Autodesk Fusion 360 part; units mm, degrees
(part 4 of 5)
  spline S20 degree 5 poles (-21.545, 23.3234) (-21.543, 23.3196) (-21.5389, 23.3119) (-21.5325, 23.3007) (-21.5232, 23.286) (-21.5109, 23.2681) (-21.4979, 23.2506) (-21.4846, 23.2333) (-21.4711, 23.2161) (-21.4574, 23.199) (-21.4435, 23.182) (-21.4295, 23.165) (-21.4152, 23.1482) (-21.4006, 23.1316) (-21.3858, 23.1152) (-21.3706, 23.0989) (-21.3553, 23.0828) (-21.3397, 23.0668) (-21.324, 23.0509) (-21.3081, 23.0351) (-21.292, 23.0195) (-21.2758, 23.0039) (-21.2594, 22.9884) (-21.2428, 22.9731) (-21.2261, 22.9579) (-21.2092, 22.9427) (-21.1921, 22.9277) (-21.1748, 22.9128) (-21.1574, 22.8981) (-21.1399, 22.8834) (-21.1222, 22.8688) (-21.1044, 22.8543) (-21.0864, 22.8399) (-21.0683, 22.8256) (-21.05, 22.8114) (-21.0316, 22.7974) (-21.0131, 22.7834) (-20.9944, 22.7695) (-20.9756, 22.7557) (-20.9567, 22.742) (-20.9377, 22.7285) (-20.9185, 22.715) (-20.8992, 22.7016) (-20.8798, 22.6883) (-20.8602, 22.6751) (-20.8406, 22.662) (-20.8208, 22.649) (-20.8009, 22.6361) (-20.7808, 22.6233) (-20.7607, 22.6106) (-20.7405, 22.598) (-20.7201, 22.5854) (-20.6996, 22.573) (-20.679, 22.5607) (-20.6583, 22.5484) (-20.6375, 22.5363) (-20.6166, 22.5243) (-20.5956, 22.5123) (-20.5744, 22.5004) (-20.5532, 22.4887) (-20.5319, 22.477) (-20.5104, 22.4654) (-20.4889, 22.454) (-20.4672, 22.4426) (-20.4455, 22.4313) (-20.4237, 22.4201) (-20.4017, 22.409) (-20.3797, 22.398) (-20.3575, 22.3871) (-20.3353, 22.3763) (-20.313, 22.3655) (-20.295, 22.357) (-20.2815, 22.3507) (-20.2725, 22.3465) (-20.268, 22.3444) knots 0 0 0 0 0 0 0.01428571 0.02857143 0.04285714 0.05714286 0.07142857 0.08571429 0.1 0.11428571 0.12857143 0.14285714 0.15714286 0.17142857 0.18571429 0.2 0.21428571 0.22857143 0.24285714 0.25714286 0.27142857 0.28571429 0.3 0.31428571 0.32857143 0.34285714 0.35714286 0.37142857 0.38571429 0.4 0.41428571 0.42857143 0.44285714 0.45714286 0.47142857 0.48571429 0.5 0.51428571 0.52857143 0.54285714 0.55714286 0.57142857 0.58571429 0.6 0.61428571 0.62857143 0.64285714 0.65714286 0.67142857 0.68571429 0.7 0.71428571 0.72857143 0.74285714 0.75714286 0.77142857 0.78571429 0.8 0.81428571 0.82857143 0.84285714 0.85714286 0.87142857 0.88571429 0.9 0.91428571 0.92857143 0.94285714 0.95714286 0.97142857 0.98571429 1 1 1 1 1 1
  line L23 (-21.545, 23.3234) -> (-21.677, 23.5776)
  arc A42 (-21.677, 23.5776) -> (-22.3193, 23.806) centre (-22.1207, 23.3471) ccw
  arc A43 (-22.5157, 23.7247) -> (-22.3193, 23.806) centre (-25, 30) ccw
  arc A44 (-22.5157, 23.7247) -> (-22.8084, 23.1089) centre (-22.3317, 23.2598) ccw
  line L24 (-22.8084, 23.1089) -> (-22.722, 22.8359)
  spline S21 degree 5 poles (-22.722, 22.8359) (-22.7207, 22.8318) (-22.7182, 22.8235) (-22.7148, 22.8109) (-22.7109, 22.794) (-22.707, 22.7727) (-22.7038, 22.7511) (-22.701, 22.7295) (-22.6984, 22.7077) (-22.696, 22.6859) (-22.6937, 22.6641) (-22.6917, 22.6422) (-22.6899, 22.6202) (-22.6885, 22.5982) (-22.6874, 22.5761) (-22.6866, 22.5539) (-22.686, 22.5316) (-22.6857, 22.5093) (-22.6856, 22.4869) (-22.6857, 22.4645) (-22.6859, 22.4421) (-22.6864, 22.4196) (-22.6871, 22.3971) (-22.6879, 22.3745) (-22.689, 22.3519) (-22.6903, 22.3292) (-22.6918, 22.3065) (-22.6934, 22.2838) (-22.6953, 22.2611) (-22.6973, 22.2383) (-22.6995, 22.2154) (-22.7018, 22.1926) (-22.7044, 22.1697) (-22.7071, 22.1468) (-22.71, 22.1239) (-22.713, 22.1009) (-22.7162, 22.0779) (-22.7196, 22.0549) (-22.7232, 22.0319) (-22.7269, 22.0088) (-22.7307, 21.9858) (-22.7348, 21.9627) (-22.7389, 21.9395) (-22.7433, 21.9164) (-22.7478, 21.8933) (-22.7524, 21.8701) (-22.7572, 21.8469) (-22.7622, 21.8237) (-22.7673, 21.8005) (-22.7725, 21.7773) (-22.7779, 21.754) (-22.7835, 21.7308) (-22.7892, 21.7075) (-22.795, 21.6842) (-22.801, 21.6609) (-22.8071, 21.6376) (-22.8134, 21.6143) (-22.8198, 21.591) (-22.8264, 21.5677) (-22.833, 21.5443) (-22.8399, 21.521) (-22.8469, 21.4977) (-22.854, 21.4743) (-22.8612, 21.451) (-22.8686, 21.4276) (-22.8762, 21.4042) (-22.8838, 21.3809) (-22.8916, 21.3575) (-22.8996, 21.3341) (-22.9076, 21.3108) (-22.9158, 21.2874) (-22.9225, 21.2687) (-22.9276, 21.2547) (-22.931, 21.2453) (-22.9327, 21.2406) knots 0 0 0 0 0 0 0.01428571 0.02857143 0.04285714 0.05714286 0.07142857 0.08571429 0.1 0.11428571 0.12857143 0.14285714 0.15714286 0.17142857 0.18571429 0.2 0.21428571 0.22857143 0.24285714 0.25714286 0.27142857 0.28571429 0.3 0.31428571 0.32857143 0.34285714 0.35714286 0.37142857 0.38571429 0.4 0.41428571 0.42857143 0.44285714 0.45714286 0.47142857 0.48571429 0.5 0.51428571 0.52857143 0.54285714 0.55714286 0.57142857 0.58571429 0.6 0.61428571 0.62857143 0.64285714 0.65714286 0.67142857 0.68571429 0.7 0.71428571 0.72857143 0.74285714 0.75714286 0.77142857 0.78571429 0.8 0.81428571 0.82857143 0.84285714 0.85714286 0.87142857 0.88571429 0.9 0.91428571 0.92857143 0.94285714 0.95714286 0.97142857 0.98571429 1 1 1 1 1 1
  arc A45 (-23.5579, 21.1163) -> (-22.9327, 21.2406) centre (-25, 30) ccw
  spline S22 degree 5 poles (-24.363, 22.5095) (-24.3627, 22.5052) (-24.3618, 22.4965) (-24.3601, 22.4837) (-24.3572, 22.4666) (-24.3527, 22.4453) (-24.3474, 22.4242) (-24.3417, 22.4031) (-24.3358, 22.382) (-24.3297, 22.361) (-24.3234, 22.3399) (-24.3169, 22.3189) (-24.3101, 22.298) (-24.303, 22.277) (-24.2956, 22.2562) (-24.2878, 22.2354) (-24.2798, 22.2146) (-24.2715, 22.1939) (-24.2631, 22.1731) (-24.2544, 22.1525) (-24.2456, 22.1318) (-24.2366, 22.1112) (-24.2274, 22.0907) (-24.2179, 22.0702) (-24.2083, 22.0497) (-24.1984, 22.0293) (-24.1884, 22.0089) (-24.1781, 21.9885) (-24.1677, 21.9682) (-24.1571, 21.9479) (-24.1464, 21.9276) (-24.1355, 21.9074) (-24.1244, 21.8873) (-24.1131, 21.8671) (-24.1016, 21.8471) (-24.09, 21.827) (-24.0783, 21.807) (-24.0663, 21.787) (-24.0542, 21.7671) (-24.042, 21.7472) (-24.0296, 21.7274) (-24.017, 21.7076) (-24.0043, 21.6878) (-23.9915, 21.6681) (-23.9785, 21.6485) (-23.9653, 21.6288) (-23.952, 21.6092) (-23.9385, 21.5897) (-23.925, 21.5702) (-23.9112, 21.5508) (-23.8973, 21.5313) (-23.8833, 21.512) (-23.8691, 21.4927) (-23.8548, 21.4734) (-23.8404, 21.4542) (-23.8258, 21.435) (-23.8111, 21.4159) (-23.7963, 21.3968) (-23.7813, 21.3777) (-23.7662, 21.3587) (-23.7509, 21.3398) (-23.7355, 21.3209) (-23.72, 21.302) (-23.7044, 21.2832) (-23.6886, 21.2645) (-23.6727, 21.2458) (-23.6567, 21.2271) (-23.6405, 21.2085) (-23.6243, 21.19) (-23.6079, 21.1715) (-23.5913, 21.153) (-23.578, 21.1383) (-23.568, 21.1273) (-23.5613, 21.12) (-23.5579, 21.1163) knots 0 0 0 0 0 0 0.01428571 0.02857143 0.04285714 0.05714286 0.07142857 0.08571429 0.1 0.11428571 0.12857143 0.14285714 0.15714286 0.17142857 0.18571429 0.2 0.21428571 0.22857143 0.24285714 0.25714286 0.27142857 0.28571429 0.3 0.31428571 0.32857143 0.34285714 0.35714286 0.37142857 0.38571429 0.4 0.41428571 0.42857143 0.44285714 0.45714286 0.47142857 0.48571429 0.5 0.51428571 0.52857143 0.54285714 0.55714286 0.57142857 0.58571429 0.6 0.61428571 0.62857143 0.64285714 0.65714286 0.67142857 0.68571429 0.7 0.71428571 0.72857143 0.74285714 0.75714286 0.77142857 0.78571429 0.8 0.81428571 0.82857143 0.84285714 0.85714286 0.87142857 0.88571429 0.9 0.91428571 0.92857143 0.94285714 0.95714286 0.97142857 0.98571429 1 1 1 1 1 1
  line L25 (-24.363, 22.5095) -> (-24.3877, 22.7948)
  arc A46 (-24.3877, 22.7948) -> (-24.8937, 23.2516) centre (-24.8858, 22.7517) ccw
  arc A47 (-25.1063, 23.2516) -> (-24.8937, 23.2516) centre (-25, 30) ccw
  arc A48 (-25.1063, 23.2516) -> (-25.6123, 22.7948) centre (-25.1142, 22.7517) ccw
  line L26 (-25.6123, 22.7948) -> (-25.637, 22.5095)
  spline S23 degree 5 poles (-25.637, 22.5095) (-25.6373, 22.5052) (-25.6382, 22.4965) (-25.6399, 22.4837) (-25.6428, 22.4666) (-25.6473, 22.4453) (-25.6526, 22.4242) (-25.6583, 22.4031) (-25.6642, 22.382) (-25.6703, 22.361) (-25.6766, 22.3399) (-25.6831, 22.3189) (-25.6899, 22.298) (-25.697, 22.277) (-25.7044, 22.2562) (-25.7122, 22.2354) (-25.7202, 22.2146) (-25.7285, 22.1939) (-25.7369, 22.1731) (-25.7456, 22.1525) (-25.7544, 22.1318) (-25.7634, 22.1112) (-25.7726, 22.0907) (-25.7821, 22.0702) (-25.7917, 22.0497) (-25.8016, 22.0293) (-25.8116, 22.0089) (-25.8219, 21.9885) (-25.8323, 21.9682) (-25.8429, 21.9479) (-25.8536, 21.9276) (-25.8645, 21.9074) (-25.8756, 21.8873) (-25.8869, 21.8671) (-25.8984, 21.8471) (-25.91, 21.827) (-25.9217, 21.807) (-25.9337, 21.787) (-25.9458, 21.7671) (-25.958, 21.7472) (-25.9704, 21.7274) (-25.983, 21.7076) (-25.9957, 21.6878) (-26.0085, 21.6681) (-26.0215, 21.6485) (-26.0347, 21.6288) (-26.048, 21.6092) (-26.0615, 21.5897) (-26.075, 21.5702) (-26.0888, 21.5508) (-26.1027, 21.5313) (-26.1167, 21.512) (-26.1309, 21.4927) (-26.1452, 21.4734) (-26.1596, 21.4542) (-26.1742, 21.435) (-26.1889, 21.4159) (-26.2037, 21.3968) (-26.2187, 21.3777) (-26.2338, 21.3587) (-26.2491, 21.3398) (-26.2645, 21.3209) (-26.28, 21.302) (-26.2956, 21.2832) (-26.3114, 21.2645) (-26.3273, 21.2458) (-26.3433, 21.2271) (-26.3595, 21.2085) (-26.3757, 21.19) (-26.3921, 21.1715) (-26.4087, 21.153) (-26.422, 21.1383) (-26.432, 21.1273) (-26.4387, 21.12) (-26.4421, 21.1163) knots 0 0 0 0 0 0 0.01428571 0.02857143 0.04285714 0.05714286 0.07142857 0.08571429 0.1 0.11428571 0.12857143 0.14285714 0.15714286 0.17142857 0.18571429 0.2 0.21428571 0.22857143 0.24285714 0.25714286 0.27142857 0.28571429 0.3 0.31428571 0.32857143 0.34285714 0.35714286 0.37142857 0.38571429 0.4 0.41428571 0.42857143 0.44285714 0.45714286 0.47142857 0.48571429 0.5 0.51428571 0.52857143 0.54285714 0.55714286 0.57142857 0.58571429 0.6 0.61428571 0.62857143 0.64285714 0.65714286 0.67142857 0.68571429 0.7 0.71428571 0.72857143 0.74285714 0.75714286 0.77142857 0.78571429 0.8 0.81428571 0.82857143 0.84285714 0.85714286 0.87142857 0.88571429 0.9 0.91428571 0.92857143 0.94285714 0.95714286 0.97142857 0.98571429 1 1 1 1 1 1
  arc A49 (-27.0673, 21.2406) -> (-26.4421, 21.1163) centre (-25, 30) ccw
  spline S24 degree 5 poles (-27.278, 22.8359) (-27.2793, 22.8318) (-27.2818, 22.8235) (-27.2852, 22.8109) (-27.2891, 22.794) (-27.293, 22.7727) (-27.2962, 22.7511) (-27.299, 22.7295) (-27.3016, 22.7077) (-27.304, 22.6859) (-27.3063, 22.6641) (-27.3083, 22.6422) (-27.3101, 22.6202) (-27.3115, 22.5982) (-27.3126, 22.5761) (-27.3134, 22.5539) (-27.314, 22.5316) (-27.3143, 22.5093) (-27.3144, 22.4869) (-27.3143, 22.4645) (-27.3141, 22.4421) (-27.3136, 22.4196) (-27.3129, 22.3971) (-27.3121, 22.3745) (-27.311, 22.3519) (-27.3097, 22.3292) (-27.3082, 22.3065) (-27.3066, 22.2838) (-27.3047, 22.2611) (-27.3027, 22.2383) (-27.3005, 22.2154) (-27.2982, 22.1926) (-27.2956, 22.1697) (-27.2929, 22.1468) (-27.29, 22.1239) (-27.287, 22.1009) (-27.2838, 22.0779) (-27.2804, 22.0549) (-27.2768, 22.0319) (-27.2731, 22.0088) (-27.2693, 21.9858) (-27.2652, 21.9627) (-27.2611, 21.9395) (-27.2567, 21.9164) (-27.2522, 21.8933) (-27.2476, 21.8701) (-27.2428, 21.8469) (-27.2378, 21.8237) (-27.2327, 21.8005) (-27.2275, 21.7773) (-27.2221, 21.754) (-27.2165, 21.7308) (-27.2108, 21.7075) (-27.205, 21.6842) (-27.199, 21.6609) (-27.1929, 21.6376) (-27.1866, 21.6143) (-27.1802, 21.591) (-27.1736, 21.5677) (-27.167, 21.5443) (-27.1601, 21.521) (-27.1531, 21.4977) (-27.146, 21.4743) (-27.1388, 21.451) (-27.1314, 21.4276) (-27.1238, 21.4042) (-27.1162, 21.3809) (-27.1084, 21.3575) (-27.1004, 21.3341) (-27.0924, 21.3108) (-27.0842, 21.2874) (-27.0775, 21.2687) (-27.0724, 21.2547) (-27.069, 21.2453) (-27.0673, 21.2406) knots 0 0 0 0 0 0 0.01428571 0.02857143 0.04285714 0.05714286 0.07142857 0.08571429 0.1 0.11428571 0.12857143 0.14285714 0.15714286 0.17142857 0.18571429 0.2 0.21428571 0.22857143 0.24285714 0.25714286 0.27142857 0.28571429 0.3 0.31428571 0.32857143 0.34285714 0.35714286 0.37142857 0.38571429 0.4 0.41428571 0.42857143 0.44285714 0.45714286 0.47142857 0.48571429 0.5 0.51428571 0.52857143 0.54285714 0.55714286 0.57142857 0.58571429 0.6 0.61428571 0.62857143 0.64285714 0.65714286 0.67142857 0.68571429 0.7 0.71428571 0.72857143 0.74285714 0.75714286 0.77142857 0.78571429 0.8 0.81428571 0.82857143 0.84285714 0.85714286 0.87142857 0.88571429 0.9 0.91428571 0.92857143 0.94285714 0.95714286 0.97142857 0.98571429 1 1 1 1 1 1
  line L27 (-27.278, 22.8359) -> (-27.1916, 23.1089)
  arc A50 (-27.1916, 23.1089) -> (-27.4843, 23.7247) centre (-27.6683, 23.2598) ccw
  arc A51 (-27.6807, 23.806) -> (-27.4843, 23.7247) centre (-25, 30) ccw
  arc A52 (-27.6807, 23.806) -> (-28.323, 23.5776) centre (-27.8793, 23.3471) ccw
  line L28 (-28.323, 23.5776) -> (-28.455, 23.3234)
  spline S25 degree 5 poles (-28.455, 23.3234) (-28.457, 23.3196) (-28.4611, 23.3119) (-28.4675, 23.3007) (-28.4768, 23.286) (-28.4891, 23.2681) (-28.5021, 23.2506) (-28.5154, 23.2333) (-28.5289, 23.2161) (-28.5426, 23.199) (-28.5565, 23.182) (-28.5705, 23.165) (-28.5848, 23.1482) (-28.5994, 23.1316) (-28.6142, 23.1152) (-28.6294, 23.0989) (-28.6447, 23.0828) (-28.6603, 23.0668) (-28.676, 23.0509) (-28.6919, 23.0351) (-28.708, 23.0195) (-28.7242, 23.0039) (-28.7406, 22.9884) (-28.7572, 22.9731) (-28.7739, 22.9579) (-28.7908, 22.9427) (-28.8079, 22.9277) (-28.8252, 22.9128) (-28.8426, 22.8981) (-28.8601, 22.8834) (-28.8778, 22.8688) (-28.8956, 22.8543) (-28.9136, 22.8399) (-28.9317, 22.8256) (-28.95, 22.8114) (-28.9684, 22.7974) (-28.9869, 22.7834) (-29.0056, 22.7695) (-29.0244, 22.7557) (-29.0433, 22.742) (-29.0623, 22.7285) (-29.0815, 22.715) (-29.1008, 22.7016) (-29.1202, 22.6883) (-29.1398, 22.6751) (-29.1594, 22.662) (-29.1792, 22.649) (-29.1991, 22.6361) (-29.2192, 22.6233) (-29.2393, 22.6106) (-29.2595, 22.598) (-29.2799, 22.5854) (-29.3004, 22.573) (-29.321, 22.5607) (-29.3417, 22.5484) (-29.3625, 22.5363) (-29.3834, 22.5243) (-29.4044, 22.5123) (-29.4256, 22.5004) (-29.4468, 22.4887) (-29.4681, 22.477) (-29.4896, 22.4654) (-29.5111, 22.454) (-29.5328, 22.4426) (-29.5545, 22.4313) (-29.5763, 22.4201) (-29.5983, 22.409) (-29.6203, 22.398) (-29.6425, 22.3871) (-29.6647, 22.3763) (-29.687, 22.3655) (-29.705, 22.357) (-29.7185, 22.3507) (-29.7275, 22.3465) (-29.732, 22.3444) knots 0 0 0 0 0 0 0.01428571 0.02857143 0.04285714 0.05714286 0.07142857 0.08571429 0.1 0.11428571 0.12857143 0.14285714 0.15714286 0.17142857 0.18571429 0.2 0.21428571 0.22857143 0.24285714 0.25714286 0.27142857 0.28571429 0.3 0.31428571 0.32857143 0.34285714 0.35714286 0.37142857 0.38571429 0.4 0.41428571 0.42857143 0.44285714 0.45714286 0.47142857 0.48571429 0.5 0.51428571 0.52857143 0.54285714 0.55714286 0.57142857 0.58571429 0.6 0.61428571 0.62857143 0.64285714 0.65714286 0.67142857 0.68571429 0.7 0.71428571 0.72857143 0.74285714 0.75714286 0.77142857 0.78571429 0.8 0.81428571 0.82857143 0.84285714 0.85714286 0.87142857 0.88571429 0.9 0.91428571 0.92857143 0.94285714 0.95714286 0.97142857 0.98571429 1 1 1 1 1 1
  arc A53 (-30.262, 22.6985) -> (-29.732, 22.3444) centre (-25, 30) ccw
  spline S26 degree 5 poles (-29.8462, 24.253) (-29.849, 24.2497) (-29.8545, 24.243) (-29.8624, 24.2327) (-29.8724, 24.2186) (-29.8842, 24.2003) (-29.8954, 24.1816) (-29.9063, 24.1627) (-29.917, 24.1436) (-29.9276, 24.1244) (-29.938, 24.1051) (-29.9483, 24.0856) (-29.9583, 24.066) (-29.9681, 24.0462) (-29.9776, 24.0262) (-29.9868, 24.006) (-29.9959, 23.9856) (-30.0047, 23.9651) (-30.0133, 23.9445) (-30.0218, 23.9238) (-30.0302, 23.9029) (-30.0384, 23.882) (-30.0464, 23.8609) (-30.0542, 23.8397) (-30.0619, 23.8184) (-30.0694, 23.797) (-30.0767, 23.7755) (-30.0838, 23.7539) (-30.0909, 23.7321) (-30.0977, 23.7103) (-30.1044, 23.6884) (-30.111, 23.6664) (-30.1174, 23.6443) (-30.1237, 23.6221) (-30.1298, 23.5998) (-30.1357, 23.5774) (-30.1416, 23.5549) (-30.1472, 23.5324) (-30.1528, 23.5097) (-30.1582, 23.487) (-30.1634, 23.4642) (-30.1686, 23.4413) (-30.1735, 23.4184) (-30.1784, 23.3953) (-30.1831, 23.3722) (-30.1877, 23.349) (-30.1921, 23.3258) (-30.1964, 23.3025) (-30.2006, 23.2791) (-30.2046, 23.2556) (-30.2085, 23.2321) (-30.2123, 23.2084) (-30.216, 23.1848) (-30.2195, 23.161) (-30.2229, 23.1372) (-30.2261, 23.1134) (-30.2292, 23.0894) (-30.2322, 23.0654) (-30.2351, 23.0414) (-30.2378, 23.0172) (-30.2405, 22.9931) (-30.2429, 22.9688) (-30.2453, 22.9445) (-30.2475, 22.9202) (-30.2497, 22.8958) (-30.2516, 22.8713) (-30.2535, 22.8468) (-30.2552, 22.8222) (-30.2568, 22.7976) (-30.2583, 22.7729) (-30.2597, 22.7482) (-30.2607, 22.7283) (-30.2614, 22.7135) (-30.2618, 22.7035) (-30.262, 22.6985) knots 0 0 0 0 0 0 0.01428571 0.02857143 0.04285714 0.05714286 0.07142857 0.08571429 0.1 0.11428571 0.12857143 0.14285714 0.15714286 0.17142857 0.18571429 0.2 0.21428571 0.22857143 0.24285714 0.25714286 0.27142857 0.28571429 0.3 0.31428571 0.32857143 0.34285714 0.35714286 0.37142857 0.38571429 0.4 0.41428571 0.42857143 0.44285714 0.45714286 0.47142857 0.48571429 0.5 0.51428571 0.52857143 0.54285714 0.55714286 0.57142857 0.58571429 0.6 0.61428571 0.62857143 0.64285714 0.65714286 0.67142857 0.68571429 0.7 0.71428571 0.72857143 0.74285714 0.75714286 0.77142857 0.78571429 0.8 0.81428571 0.82857143 0.84285714 0.85714286 0.87142857 0.88571429 0.9 0.91428571 0.92857143 0.94285714 0.95714286 0.97142857 0.98571429 1 1 1 1 1 1
  line L29 (-29.8462, 24.253) -> (-29.6619, 24.4722)
  arc A54 (-29.6619, 24.4722) -> (-29.6967, 25.153) centre (-30.0446, 24.794) ccw
  arc A55 (-29.847, 25.3033) -> (-29.6967, 25.153) centre (-25, 30) ccw
  arc A56 (-29.847, 25.3033) -> (-30.5278, 25.3381) centre (-30.206, 24.9554) ccw
  line L30 (-30.5278, 25.3381) -> (-30.747, 25.1538)
  spline S27 degree 5 poles (-30.747, 25.1538) (-30.7503, 25.151) (-30.757, 25.1455) (-30.7673, 25.1376) (-30.7814, 25.1276) (-30.7997, 25.1158) (-30.8184, 25.1046) (-30.8373, 25.0937) (-30.8564, 25.083) (-30.8756, 25.0724) (-30.8949, 25.062) (-30.9144, 25.0517) (-30.934, 25.0417) (-30.9538, 25.0319) (-30.9738, 25.0224) (-30.994, 25.0132) (-31.0144, 25.0041) (-31.0349, 24.9953) (-31.0555, 24.9867) (-31.0762, 24.9782) (-31.0971, 24.9698) (-31.118, 24.9616) (-31.1391, 24.9536) (-31.1603, 24.9458) (-31.1816, 24.9381) (-31.203, 24.9306) (-31.2245, 24.9233) (-31.2461, 24.9162) (-31.2679, 24.9091) (-31.2897, 24.9023) (-31.3116, 24.8956) (-31.3336, 24.889) (-31.3557, 24.8826) (-31.3779, 24.8763) (-31.4002, 24.8702) (-31.4226, 24.8643) (-31.4451, 24.8584) (-31.4676, 24.8528) (-31.4903, 24.8472) (-31.513, 24.8418) (-31.5358, 24.8366) (-31.5587, 24.8314) (-31.5816, 24.8265) (-31.6047, 24.8216) (-31.6278, 24.8169) (-31.651, 24.8123) (-31.6742, 24.8079) (-31.6975, 24.8036) (-31.7209, 24.7994) (-31.7444, 24.7954) (-31.7679, 24.7915) (-31.7916, 24.7877) (-31.8152, 24.784) (-31.839, 24.7805) (-31.8628, 24.7771) (-31.8866, 24.7739) (-31.9106, 24.7708) (-31.9346, 24.7678) (-31.9586, 24.7649) (-31.9828, 24.7622) (-32.0069, 24.7595) (-32.0312, 24.7571) (-32.0555, 24.7547) (-32.0798, 24.7525) (-32.1042, 24.7503) (-32.1287, 24.7484) (-32.1532, 24.7465) (-32.1778, 24.7448) (-32.2024, 24.7432) (-32.2271, 24.7417) (-32.2518, 24.7403) (-32.2717, 24.7393) (-32.2865, 24.7386) (-32.2965, 24.7382) (-32.3015, 24.738) knots 0 0 0 0 0 0 0.01428571 0.02857143 0.04285714 0.05714286 0.07142857 0.08571429 0.1 0.11428571 0.12857143 0.14285714 0.15714286 0.17142857 0.18571429 0.2 0.21428571 0.22857143 0.24285714 0.25714286 0.27142857 0.28571429 0.3 0.31428571 0.32857143 0.34285714 0.35714286 0.37142857 0.38571429 0.4 0.41428571 0.42857143 0.44285714 0.45714286 0.47142857 0.48571429 0.5 0.51428571 0.52857143 0.54285714 0.55714286 0.57142857 0.58571429 0.6 0.61428571 0.62857143 0.64285714 0.65714286 0.67142857 0.68571429 0.7 0.71428571 0.72857143 0.74285714 0.75714286 0.77142857 0.78571429 0.8 0.81428571 0.82857143 0.84285714 0.85714286 0.87142857 0.88571429 0.9 0.91428571 0.92857143 0.94285714 0.95714286 0.97142857 0.98571429 1 1 1 1 1 1
  arc A57 (-32.6556, 25.268) -> (-32.3015, 24.738) centre (-25, 30) ccw
  spline S28 degree 5 poles (-31.6766, 26.545) (-31.6804, 26.543) (-31.6881, 26.5389) (-31.6993, 26.5325) (-31.714, 26.5232) (-31.7319, 26.5109) (-31.7494, 26.4979) (-31.7667, 26.4846) (-31.7839, 26.4711) (-31.801, 26.4574) (-31.818, 26.4435) (-31.835, 26.4295) (-31.8518, 26.4152) (-31.8684, 26.4006) (-31.8848, 26.3858) (-31.9011, 26.3706) (-31.9172, 26.3553) (-31.9332, 26.3397) (-31.9491, 26.324) (-31.9649, 26.3081) (-31.9805, 26.292) (-31.9961, 26.2758) (-32.0116, 26.2594) (-32.0269, 26.2428) (-32.0421, 26.2261) (-32.0573, 26.2092) (-32.0723, 26.1921) (-32.0872, 26.1748) (-32.1019, 26.1574) (-32.1166, 26.1399) (-32.1312, 26.1222) (-32.1457, 26.1044) (-32.1601, 26.0864) (-32.1744, 26.0683) (-32.1886, 26.05) (-32.2026, 26.0316) (-32.2166, 26.0131) (-32.2305, 25.9944) (-32.2443, 25.9756) (-32.258, 25.9567) (-32.2715, 25.9377) (-32.285, 25.9185) (-32.2984, 25.8992) (-32.3117, 25.8798) (-32.3249, 25.8602) (-32.338, 25.8406) (-32.351, 25.8208) (-32.3639, 25.8009) (-32.3767, 25.7808) (-32.3894, 25.7607) (-32.402, 25.7405) (-32.4146, 25.7201) (-32.427, 25.6996) (-32.4393, 25.679) (-32.4516, 25.6583) (-32.4637, 25.6375) (-32.4757, 25.6166) (-32.4877, 25.5956) (-32.4996, 25.5744) (-32.5113, 25.5532) (-32.523, 25.5319) (-32.5346, 25.5104) (-32.546, 25.4889) (-32.5574, 25.4672) (-32.5687, 25.4455) (-32.5799, 25.4237) (-32.591, 25.4017) (-32.602, 25.3797) (-32.6129, 25.3575) (-32.6237, 25.3353) (-32.6345, 25.313) (-32.643, 25.295) (-32.6493, 25.2815) (-32.6535, 25.2725) (-32.6556, 25.268) knots 0 0 0 0 0 0 0.01428571 0.02857143 0.04285714 0.05714286 0.07142857 0.08571429 0.1 0.11428571 0.12857143 0.14285714 0.15714286 0.17142857 0.18571429 0.2 0.21428571 0.22857143 0.24285714 0.25714286 0.27142857 0.28571429 0.3 0.31428571 0.32857143 0.34285714 0.35714286 0.37142857 0.38571429 0.4 0.41428571 0.42857143 0.44285714 0.45714286 0.47142857 0.48571429 0.5 0.51428571 0.52857143 0.54285714 0.55714286 0.57142857 0.58571429 0.6 0.61428571 0.62857143 0.64285714 0.65714286 0.67142857 0.68571429 0.7 0.71428571 0.72857143 0.74285714 0.75714286 0.77142857 0.78571429 0.8 0.81428571 0.82857143 0.84285714 0.85714286 0.87142857 0.88571429 0.9 0.91428571 0.92857143 0.94285714 0.95714286 0.97142857 0.98571429 1 1 1 1 1 1
  line L31 (-31.6766, 26.545) -> (-31.4224, 26.677)
  arc A58 (-31.4224, 26.677) -> (-31.194, 27.3193) centre (-31.6529, 27.1207) ccw
  arc A59 (-31.2753, 27.5157) -> (-31.194, 27.3193) centre (-25, 30) ccw
  arc A60 (-31.2753, 27.5157) -> (-31.8911, 27.8084) centre (-31.7402, 27.3317) ccw
  line L32 (-31.8911, 27.8084) -> (-32.1641, 27.722)
  spline S29 degree 5 poles (-32.1641, 27.722) (-32.1682, 27.7207) (-32.1765, 27.7182) (-32.1891, 27.7148) (-32.206, 27.7109) (-32.2273, 27.707) (-32.2489, 27.7038) (-32.2705, 27.701) (-32.2923, 27.6984) (-32.3141, 27.696) (-32.3359, 27.6937) (-32.3578, 27.6917) (-32.3798, 27.6899) (-32.4018, 27.6885) (-32.4239, 27.6874) (-32.4461, 27.6866) (-32.4684, 27.686) (-32.4907, 27.6857) (-32.5131, 27.6856) (-32.5355, 27.6857) (-32.5579, 27.6859) (-32.5804, 27.6864) (-32.6029, 27.6871) (-32.6255, 27.6879) (-32.6481, 27.689) (-32.6708, 27.6903) (-32.6935, 27.6918) (-32.7162, 27.6934) (-32.7389, 27.6953) (-32.7617, 27.6973) (-32.7846, 27.6995) (-32.8074, 27.7018) (-32.8303, 27.7044) (-32.8532, 27.7071) (-32.8761, 27.71) (-32.8991, 27.713) (-32.9221, 27.7162) (-32.9451, 27.7196) (-32.9681, 27.7232) (-32.9912, 27.7269) (-33.0142, 27.7307) (-33.0373, 27.7348) (-33.0605, 27.7389) (-33.0836, 27.7433) (-33.1067, 27.7478) (-33.1299, 27.7524) (-33.1531, 27.7572) (-33.1763, 27.7622) (-33.1995, 27.7673) (-33.2227, 27.7725) (-33.246, 27.7779) (-33.2692, 27.7835) (-33.2925, 27.7892) (-33.3158, 27.795) (-33.3391, 27.801) (-33.3624, 27.8071) (-33.3857, 27.8134) (-33.409, 27.8198) (-33.4323, 27.8264) (-33.4557, 27.833) (-33.479, 27.8399) (-33.5023, 27.8469) (-33.5257, 27.854) (-33.549, 27.8612) (-33.5724, 27.8686) (-33.5958, 27.8762) (-33.6191, 27.8838) (-33.6425, 27.8916) (-33.6659, 27.8996) (-33.6892, 27.9076) (-33.7126, 27.9158) (-33.7313, 27.9225) (-33.7453, 27.9276) (-33.7547, 27.931) (-33.7594, 27.9327) knots 0 0 0 0 0 0 0.01428571 0.02857143 0.04285714 0.05714286 0.07142857 0.08571429 0.1 0.11428571 0.12857143 0.14285714 0.15714286 0.17142857 0.18571429 0.2 0.21428571 0.22857143 0.24285714 0.25714286 0.27142857 0.28571429 0.3 0.31428571 0.32857143 0.34285714 0.35714286 0.37142857 0.38571429 0.4 0.41428571 0.42857143 0.44285714 0.45714286 0.47142857 0.48571429 0.5 0.51428571 0.52857143 0.54285714 0.55714286 0.57142857 0.58571429 0.6 0.61428571 0.62857143 0.64285714 0.65714286 0.67142857 0.68571429 0.7 0.71428571 0.72857143 0.74285714 0.75714286 0.77142857 0.78571429 0.8 0.81428571 0.82857143 0.84285714 0.85714286 0.87142857 0.88571429 0.9 0.91428571 0.92857143 0.94285714 0.95714286 0.97142857 0.98571429 1 1 1 1 1 1
  arc A61 (-33.8837, 28.5579) -> (-33.7594, 27.9327) centre (-25, 30) ccw
  spline S30 degree 5 poles (-32.4905, 29.363) (-32.4948, 29.3627) (-32.5035, 29.3618) (-32.5163, 29.3601) (-32.5334, 29.3572) (-32.5547, 29.3527) (-32.5758, 29.3474) (-32.5969, 29.3417) (-32.618, 29.3358) (-32.639, 29.3297) (-32.6601, 29.3234) (-32.6811, 29.3169) (-32.702, 29.3101) (-32.723, 29.303) (-32.7438, 29.2956) (-32.7646, 29.2878) (-32.7854, 29.2798) (-32.8061, 29.2715) (-32.8269, 29.2631) (-32.8475, 29.2544) (-32.8682, 29.2456) (-32.8888, 29.2366) (-32.9093, 29.2274) (-32.9298, 29.2179) (-32.9503, 29.2083) (-32.9707, 29.1984) (-32.9911, 29.1884) (-33.0115, 29.1781) (-33.0318, 29.1677) (-33.0521, 29.1571) (-33.0724, 29.1464) (-33.0926, 29.1355) (-33.1127, 29.1244) (-33.1329, 29.1131) (-33.1529, 29.1016) (-33.173, 29.09) (-33.193, 29.0783) (-33.213, 29.0663) (-33.2329, 29.0542) (-33.2528, 29.042) (-33.2726, 29.0296) (-33.2924, 29.017) (-33.3122, 29.0043) (-33.3319, 28.9915) (-33.3515, 28.9785) (-33.3712, 28.9653) (-33.3908, 28.952) (-33.4103, 28.9385) (-33.4298, 28.925) (-33.4492, 28.9112) (-33.4687, 28.8973) (-33.488, 28.8833) (-33.5073, 28.8691) (-33.5266, 28.8548) (-33.5458, 28.8404) (-33.565, 28.8258) (-33.5841, 28.8111) (-33.6032, 28.7963) (-33.6223, 28.7813) (-33.6413, 28.7662) (-33.6602, 28.7509) (-33.6791, 28.7355) (-33.698, 28.72) (-33.7168, 28.7044) (-33.7355, 28.6886) (-33.7542, 28.6727) (-33.7729, 28.6567) (-33.7915, 28.6405) (-33.81, 28.6243) (-33.8285, 28.6079) (-33.847, 28.5913) (-33.8617, 28.578) (-33.8727, 28.568) (-33.88, 28.5613) (-33.8837, 28.5579) knots 0 0 0 0 0 0 0.01428571 0.02857143 0.04285714 0.05714286 0.07142857 0.08571429 0.1 0.11428571 0.12857143 0.14285714 0.15714286 0.17142857 0.18571429 0.2 0.21428571 0.22857143 0.24285714 0.25714286 0.27142857 0.28571429 0.3 0.31428571 0.32857143 0.34285714 0.35714286 0.37142857 0.38571429 0.4 0.41428571 0.42857143 0.44285714 0.45714286 0.47142857 0.48571429 0.5 0.51428571 0.52857143 0.54285714 0.55714286 0.57142857 0.58571429 0.6 0.61428571 0.62857143 0.64285714 0.65714286 0.67142857 0.68571429 0.7 0.71428571 0.72857143 0.74285714 0.75714286 0.77142857 0.78571429 0.8 0.81428571 0.82857143 0.84285714 0.85714286 0.87142857 0.88571429 0.9 0.91428571 0.92857143 0.94285714 0.95714286 0.97142857 0.98571429 1 1 1 1 1 1
  line L33 (-32.4905, 29.363) -> (-32.2052, 29.3877)
  arc A62 (-32.2052, 29.3877) -> (-31.7484, 29.8937) centre (-32.2483, 29.8858) ccw
  arc A63 (-31.7484, 30.1063) -> (-31.7484, 29.8937) centre (-25, 30) ccw
  arc A64 (-31.7484, 30.1063) -> (-32.2052, 30.6123) centre (-32.2483, 30.1142) ccw
  line L34 (-32.2052, 30.6123) -> (-32.4905, 30.637)
  spline S31 degree 5 poles (-32.4905, 30.637) (-32.4948, 30.6373) (-32.5035, 30.6382) (-32.5163, 30.6399) (-32.5334, 30.6428) (-32.5547, 30.6473) (-32.5758, 30.6526) (-32.5969, 30.6583) (-32.618, 30.6642) (-32.639, 30.6703) (-32.6601, 30.6766) (-32.6811, 30.6831) (-32.702, 30.6899) (-32.723, 30.697) (-32.7438, 30.7044) (-32.7646, 30.7122) (-32.7854, 30.7202) (-32.8061, 30.7285) (-32.8269, 30.7369) (-32.8475, 30.7456) (-32.8682, 30.7544) (-32.8888, 30.7634) (-32.9093, 30.7726) (-32.9298, 30.7821) (-32.9503, 30.7917) (-32.9707, 30.8016) (-32.9911, 30.8116) (-33.0115, 30.8219) (-33.0318, 30.8323) (-33.0521, 30.8429) (-33.0724, 30.8536) (-33.0926, 30.8645) (-33.1127, 30.8756) (-33.1329, 30.8869) (-33.1529, 30.8984) (-33.173, 30.91) (-33.193, 30.9217) (-33.213, 30.9337) (-33.2329, 30.9458) (-33.2528, 30.958) (-33.2726, 30.9704) (-33.2924, 30.983) (-33.3122, 30.9957) (-33.3319, 31.0085) (-33.3515, 31.0215) (-33.3712, 31.0347) (-33.3908, 31.048) (-33.4103, 31.0615) (-33.4298, 31.075) (-33.4492, 31.0888) (-33.4687, 31.1027) (-33.488, 31.1167) (-33.5073, 31.1309) (-33.5266, 31.1452) (-33.5458, 31.1596) (-33.565, 31.1742) (-33.5841, 31.1889) (-33.6032, 31.2037) (-33.6223, 31.2187) (-33.6413, 31.2338) (-33.6602, 31.2491) (-33.6791, 31.2645) (-33.698, 31.28) (-33.7168, 31.2956) (-33.7355, 31.3114) (-33.7542, 31.3273) (-33.7729, 31.3433) (-33.7915, 31.3595) (-33.81, 31.3757) (-33.8285, 31.3921) (-33.847, 31.4087) (-33.8617, 31.422) (-33.8727, 31.432) (-33.88, 31.4387) (-33.8837, 31.4421) knots 0 0 0 0 0 0 0.01428571 0.02857143 0.04285714 0.05714286 0.07142857 0.08571429 0.1 0.11428571 0.12857143 0.14285714 0.15714286 0.17142857 0.18571429 0.2 0.21428571 0.22857143 0.24285714 0.25714286 0.27142857 0.28571429 0.3 0.31428571 0.32857143 0.34285714 0.35714286 0.37142857 0.38571429 0.4 0.41428571 0.42857143 0.44285714 0.45714286 0.47142857 0.48571429 0.5 0.51428571 0.52857143 0.54285714 0.55714286 0.57142857 0.58571429 0.6 0.61428571 0.62857143 0.64285714 0.65714286 0.67142857 0.68571429 0.7 0.71428571 0.72857143 0.74285714 0.75714286 0.77142857 0.78571429 0.8 0.81428571 0.82857143 0.84285714 0.85714286 0.87142857 0.88571429 0.9 0.91428571 0.92857143 0.94285714 0.95714286 0.97142857 0.98571429 1 1 1 1 1 1
  arc A65 (-33.7594, 32.0673) -> (-33.8837, 31.4421) centre (-25, 30) ccw
  spline S32 degree 5 poles (-32.1641, 32.278) (-32.1682, 32.2793) (-32.1765, 32.2818) (-32.1891, 32.2852) (-32.206, 32.2891) (-32.2273, 32.293) (-32.2489, 32.2962) (-32.2705, 32.299) (-32.2923, 32.3016) (-32.3141, 32.304) (-32.3359, 32.3063) (-32.3578, 32.3083) (-32.3798, 32.3101) (-32.4018, 32.3115) (-32.4239, 32.3126) (-32.4461, 32.3134) (-32.4684, 32.314) (-32.4907, 32.3143) (-32.5131, 32.3144) (-32.5355, 32.3143) (-32.5579, 32.3141) (-32.5804, 32.3136) (-32.6029, 32.3129) (-32.6255, 32.3121) (-32.6481, 32.311) (-32.6708, 32.3097) (-32.6935, 32.3082) (-32.7162, 32.3066) (-32.7389, 32.3047) (-32.7617, 32.3027) (-32.7846, 32.3005) (-32.8074, 32.2982) (-32.8303, 32.2956) (-32.8532, 32.2929) (-32.8761, 32.29) (-32.8991, 32.287) (-32.9221, 32.2838) (-32.9451, 32.2804) (-32.9681, 32.2768) (-32.9912, 32.2731) (-33.0142, 32.2693) (-33.0373, 32.2652) (-33.0605, 32.2611) (-33.0836, 32.2567) (-33.1067, 32.2522) (-33.1299, 32.2476) (-33.1531, 32.2428) (-33.1763, 32.2378) (-33.1995, 32.2327) (-33.2227, 32.2275) (-33.246, 32.2221) (-33.2692, 32.2165) (-33.2925, 32.2108) (-33.3158, 32.205) (-33.3391, 32.199) (-33.3624, 32.1929) (-33.3857, 32.1866) (-33.409, 32.1802) (-33.4323, 32.1736) (-33.4557, 32.167) (-33.479, 32.1601) (-33.5023, 32.1531) (-33.5257, 32.146) (-33.549, 32.1388) (-33.5724, 32.1314) (-33.5958, 32.1238) (-33.6191, 32.1162) (-33.6425, 32.1084) (-33.6659, 32.1004) (-33.6892, 32.0924) (-33.7126, 32.0842) (-33.7313, 32.0775) (-33.7453, 32.0724) (-33.7547, 32.069) (-33.7594, 32.0673) knots 0 0 0 0 0 0 0.01428571 0.02857143 0.04285714 0.05714286 0.07142857 0.08571429 0.1 0.11428571 0.12857143 0.14285714 0.15714286 0.17142857 0.18571429 0.2 0.21428571 0.22857143 0.24285714 0.25714286 0.27142857 0.28571429 0.3 0.31428571 0.32857143 0.34285714 0.35714286 0.37142857 0.38571429 0.4 0.41428571 0.42857143 0.44285714 0.45714286 0.47142857 0.48571429 0.5 0.51428571 0.52857143 0.54285714 0.55714286 0.57142857 0.58571429 0.6 0.61428571 0.62857143 0.64285714 0.65714286 0.67142857 0.68571429 0.7 0.71428571 0.72857143 0.74285714 0.75714286 0.77142857 0.78571429 0.8 0.81428571 0.82857143 0.84285714 0.85714286 0.87142857 0.88571429 0.9 0.91428571 0.92857143 0.94285714 0.95714286 0.97142857 0.98571429 1 1 1 1 1 1
  line L35 (-32.1641, 32.278) -> (-31.8911, 32.1916)
  arc A66 (-31.8911, 32.1916) -> (-31.2753, 32.4843) centre (-31.7402, 32.6683) ccw
  line L36 (-32.375, 45.0877) -> (-32.375, 8.0877) construction
  line L37 (-34.25, 45.0877) -> (-34.25, 8.0877) construction
  circle A67 centre (-25, 30) radius 4.475
  line L38 (-47, 0) -> (-3, 0)
  line L39 (-3, 0) -> (-3, 60)
  line L40 (-3, 60) -> (-47, 60)
  line L41 (-47, 60) -> (-47, 0)
  circle A68 centre (-33, 30) radius 0.7496 construction
  circle A69 centre (-33, 30) radius 0.6996 construction
  line L42 (-32.375, 30.5171) -> (-34.25, 31.1995)
  line L43 (-34.25, 31.1995) -> (-34.25, 30)
  line L44 (-32.375, 30.5171) -> (-32.375, 30)
  line L45 (-32.375, 29.4829) -> (-32.375, 30)
  line L46 (-32.375, 29.4829) -> (-34.25, 28.8005)
  line L47 (-34.25, 28.8005) -> (-34.25, 30)
  circle A70 centre (-10, 45) radius 2.45
  circle A71 centre (-40, 15) radius 2.45
  point P0 (-25, 30)
  point P1 (-32.1702, 27.7201)
  point P2 (-32.7436, 29.2956)
  dimension "d51" = 16
  dimension "d52" = 20
  dimension "d78" = 0.625
  dimension "d79" = 1.25
  dimension "d82" = 0.05
  dimension "d84" = 20
  constraint vertical L0
  constraint coincident P0 A0.centre
  constraint tangent L0 A0
  constraint coincident L0 L2.start
  constraint coincident A0 L2.start
  constraint coincident L2 P1
  constraint coincident S29 P1
  constraint coincident S30 P2
  constraint coincident L2 P2
  constraint coincident L2.start A68.centre
  constraint coincident P2 A68
  constraint coincident L36 L42.start
  constraint coincident L37 L42.end
  constraint tangent A69 L42
  constraint coincident L37 L43.end
  constraint coincident L1 L43.end
  constraint perpendicular L1 L43
  constraint coincident L36 L44.end
  constraint coincident L1 L44.end
  constraint perpendicular L1 L44
  constraint symmetric L1 L42.start L45.start
  constraint symmetric L1 L42.end L46.end
  constraint symmetric L1 L43.end L47.end
  constraint symmetric L1 L44.end L45.end
  measures "d51" diameter of A0
  measures "d52" angle of L0 L2
  measures "d84" angle of L1 L42
extrude "Extrude8" add sketch "Rack Tooth" along normal blind 5 separate body contours L42 L43 L44 L45 L46 L47 makes body 3
pattern_linear "R-Pattern1" count 17 spacing 3.4361 along (0, 0, -1) both ways of bodies 3 makes body 4 at (33, 8.6667, 42.9999) makes body 5 at (33, 8.6667, 39.5638) makes body 6 at (33, 8.6667, 36.1277) makes body 7 at (33, 8.6667, 32.6916) makes body 8 at (33, 8.6667, 25.8193) makes body 9 at (33, 8.6667, 22.3832) makes body 10 at (33, 8.6667, 18.9471) makes body 11 at (33, 8.6667, 15.511) makes body 12 at (33, 8.6667, 12.0749) makes body 13 at (33, 8.6667, 56.7444) makes body 14 at (33, 8.6667, 53.3083) makes body 15 at (33, 8.6667, 49.8722) makes body 16 at (33, 8.6667, 46.436) makes body 17 at (33, 8.6667, 8.6388) makes body 18 at (33, 8.6667, 5.2026) makes body 19 at (33, 8.6667, 1.7665)
sketch "Rack Base" plane through (0, 7, 0) normal (0, 1, 0) x (-1, 0, 0)
  line L0 (-34.2462, 60) -> (-47, 60)
  line L1 (-47, 60) -> (-47, 0)
  line L2 (-34.2462, 0) -> (-34.2462, 60)
  line L3 (-47, 60) -> (-3, 60)
  line L4 (-47, 60) -> (-3, 60)
  line L5 (-50, 0) -> (-50, -3)
  line L6 (-50, -3) -> (0, -3)
  line L7 (0, -3) -> (0, 0)
  line L8 (0, 0) -> (-34.2462, 0)
  line L9 (-47, 0) -> (-50, 0)
  line L10 (-47, 0) -> (-34.2462, 0)
  line L11 (-45, 45) -> (-45, 44.998)
  circle A0 centre (-40, 15) radius 5
  line L12 (-35, 15.0033) -> (-35, 15)
  circle A1 centre (-40, 15) radius 2.45
  arc A2 (-45, 45.002) -> (-45, 44.998) centre (-40, 45) ccw
  line L13 (-47, 60) -> (-47, 0)
  arc A3 (-42.45, 19.3586) -> (-37.55, 19.3586) centre (-40, 15) ccw
  point P0 (-50, 0)
  point P1 (-37.55, 15)
  point P2 (-42.45, 15)
  dimension "d91" = 3
  dimension "d98" = 12.7538
  constraint perpendicular L0 L1
  constraint parallel L1 L2
  constraint coincident L0.end L4
  constraint coincident L0.start L4
  constraint perpendicular L5 L6
  constraint parallel L5 L7
  constraint parallel L6 L8
  constraint coincident P0 L5.start
  constraint collinear L8 L9
  constraint perpendicular L2 L10
  constraint coincident A0 L12.end
  constraint tangent L12 A2
  constraint concentric A1 A3
  constraint coincident A0 A3.start
  constraint coincident A0 A3.end
  constraint coincident A0 L12.start
  measures "d91" distance of P0 L5.end
  measures "d98" distance of L2 L13
extrude "Extrude9" add sketch "Rack Base" along normal blind 8 contours L0 L1 L2 L3 L4 L10 L13 | A0 L12 A3 | A1 bodies 3 13 14 15 16 4 5 6 7 8 9 10 11 12 17 18 19
extrude "Extrude10" add sketch "Rack Base" along normal blind 60 contours L5 L6 L7 L8 L9 L10 bodies 3
combine "Combine1" operation cut target body 3 tool bodies 1 keep tools
sketch "Rack Top" plane through (0, 17.2, 0) normal (0, 1, 0) x (-1, 0, 0)
  line L0 (-42.14, 60) -> (-42.14, 0)
  line L1 (-42.14, 0) -> (-34.2462, 0)
  line L2 (-34.2462, 0) -> (-34.2462, 60)
  line L3 (-34.2462, 60) -> (-42.14, 60)
  circle A0 centre (-40, 15) radius 2.45
  circle A1 centre (-40, 15) radius 5
  circle A2 centre (-40, 15) radius 2.45
  arc A3 (-42.45, 19.3586) -> (-37.55, 19.3586) centre (-40, 15) ccw
  circle A4 centre (-40, 45) radius 2.45
  circle A5 centre (-40, 45) radius 5
  line L4 (-35, 45) -> (-45, 45) construction
  line L5 (-35, 15.0033) -> (-45, 15.0073) construction
  line L6 (-35, 45) -> (-35, 15.0033)
  line L7 (-45, 15.0073) -> (-45, 45)
  line L8 (-37.55, 15) -> (-37.55, 45)
  line L9 (-42.45, 45) -> (-42.45, 15)
  line L10 (-47, 0) -> (-3, 0)
  line L11 (-3, 60) -> (-47, 60)
  line L12 (-25, 0) -> (-25, 60) construction
  line L13 (-15, 45) -> (-5, 45) construction
  line L14 (-15, 15.0033) -> (-5, 15.0073) construction
  line L15 (-15, 45) -> (-15, 15.0033)
  line L16 (-5, 15.0073) -> (-5, 45)
  line L17 (-12.45, 15) -> (-12.45, 45)
  line L18 (-7.55, 45) -> (-7.55, 15)
  circle A6 centre (-10, 15) radius 5
  circle A7 centre (-10, 15) radius 2.45
  circle A8 centre (-10, 15) radius 2.45
  arc A9 (-12.45, 19.3586) -> (-7.55, 19.3586) centre (-10, 15) ccw
  circle A10 centre (-10, 45) radius 2.45
  circle A11 centre (-10, 45) radius 5
  line L19 (-8, 0) -> (0, 0)
  line L20 (0, 0) -> (0, 60)
  line L21 (0, 60) -> (-8, 60)
  line L22 (-8, 60) -> (-8, 0)
  point P0 (-40, 15)
  point P1 (-40, 45)
  point P2 (-45, 45)
  point P3 (-35, 15.0033)
  point P4 (-35, 15.0033)
  point P5 (-45, 15.0073)
  point P6 (-35, 45)
  point P7 (-45, 45)
  point P8 (-37.55, 45)
  point P9 (-42.45, 45)
  point P10 (-42.45, 15)
  point P11 (-42.45, 15)
  point P12 (-37.55, 15)
  point P13 (-37.55, 15)
  point P14 (-10, 15)
  point P15 (-15, 45)
  point P16 (-10, 45)
  point P17 (-5, 45)
  point P18 (-15, 15.0033)
  point P19 (-15, 15.0033)
  point P20 (-5, 15.0073)
  point P21 (-5, 45)
  point P22 (-12.45, 45)
  point P23 (-7.55, 45)
  point P24 (-7.55, 15)
  point P25 (-7.55, 15)
  point P26 (-12.45, 15)
  point P27 (-12.45, 15)
  constraint coincident P0 A0.centre
  constraint equal A0 A2
  constraint equal A1 A3
  constraint coincident P1 A4.centre
  constraint equal A0 A4
  constraint equal A1 A5
  constraint coincident A5 P6
  constraint coincident P7 P2
  constraint perpendicular L0 L4
  constraint coincident P4 P3
  constraint coincident A1 P5
  constraint coincident P5 L5.end
  constraint coincident P6 L4.start
  constraint coincident A4 P8
  constraint coincident L4 P8
  constraint coincident A4 P9
  constraint coincident L4 P9
  constraint coincident P11 P10
  constraint coincident P13 P12
  constraint coincident P8 L8.end
  constraint coincident P9 L9.start
  constraint midpoint L10 L12.start
  constraint midpoint L11 L12.end
  constraint symmetric A0 L12 A8
  constraint symmetric P0 L12 P14
  constraint symmetric A1 L12 A6
  constraint symmetric A2 L12 A7
  constraint symmetric A3.start L12 A9.end
  constraint symmetric A3.end L12 A9.start
  constraint symmetric A3 L12 A9
  constraint symmetric A4 L12 A10
  constraint symmetric P1 L12 P16
  constraint symmetric A5 L12 A11
  constraint symmetric P7 L12 P21
  constraint symmetric P6 L12 P15
  constraint symmetric P4 L12 P19
  constraint symmetric P4 L12 P18
  constraint symmetric P5 L12 L14.end
  constraint symmetric P5 L12 P20
  constraint symmetric P8 L12 P22
  constraint symmetric P9 L12 P23
  constraint symmetric P11 L12 P25
  constraint symmetric P13 L12 P27
extrude "Extrude12" cut sketch "Rack Top" against normal up to surface (10.2 mm away) contours L0 A4 | L0 A4 | L0 A4 A5 L8 | L0 A4 A5 L9 | L0 A1 A5 L8 | L0 A1 A5 L9 | L0 A0 A1 A2 L8 | L0 A0 A1 A2 L9 | L0 A0 A2 | L0 A0 A2 picked at (-41.4807, 41.1321) picked at (-42.288, 42.8456) bodies 3
extrude "Extrude13" cut sketch "Rack Top" against normal up to surface (8.2 mm away) contours L0 A4 A5 L8 | L0 A4 A5 L9 | A1 A3 A5 L6 L8 | A1 A3 A5 L7 L9 | L0 A0 A1 A2 A3 L8 | L0 A0 A1 A2 A3 L9 picked at (-41.4688, 48.8716) picked at (-43.6413, 46.9734) bodies 3
extrude "Extrude15" cut sketch "Rack Top" against normal up to surface (10.2 mm away) contours L0 A0 A1 A2 A3 L8 | L0 A0 A1 A2 A3 L9 | L17 A10 A11 L22 | L18 A10 A11 L22 | L0 A0 A1 A2 L8 | L0 A0 A1 A2 L9 | A10 L22 | A10 L22 | L0 A0 A2 | L0 A0 A2 | L18 A10 A11 L22 | L17 A10 A11 L22 bodies 1
extrude "Extrude17" add sketch "Base Top" along normal blind 2 contours A4 L14 L15 L16 | A4 L13 L14 L16 | A2 A4 L13 L14 | A2 A4 L14 L15 | A5 L17 L18 L20 | A3 A5 L17 L18 | A5 L18 L19 L20 | A3 A5 L18 L19 picked at (-40.877, 10.9511) picked at (-42.2029, 12.6892) picked at (-9.123, 49.0489) picked at (-7.7971, 47.3108) bodies 1
sketch "Rack Side" plane through (0, 0, 60) normal (0, 0, 1) x (1, 0, 0)
  line L0 (47, 8.0593) -> (42.14, 15)
  line L1 (42.14, 15) -> (34.2462, 15)
  line L2 (34.2462, 15) -> (34.2462, 7)
  line L3 (34.2462, 7) -> (47, 7)
  line L4 (47, 7) -> (47, 8.0593)
  line L5 (42.5, 7) -> (42.5, 9.1)
  line L6 (42.5, 9.1) -> (37.5, 9.1)
  line L7 (37.5, 9.1) -> (37.5, 7)
  line L8 (37.5, 7) -> (42.5, 7)
  dimension "d129" = 2.1
  dimension "d130" = 5
  dimension "d131" = 4.5
  constraint perpendicular L5 L6
  constraint parallel L5 L7
  constraint parallel L6 L8
  constraint perpendicular L3 L5
  constraint coincident L3 L5.start
  measures "d129" distance of L5.start L5.end
  measures "d130" distance of L5.start L7.end
  measures "d131" distance of L4 L5
combine "Combine2" operation cut target body 3 tool bodies 1 keep tools
extrude "Extrude19" cut sketch "Base Top" against normal up to surface (7 mm away) contours A6 | A8 bodies 1
extrude "Extrude20" cut sketch "Base Top" against normal blind 3 contours A7 | A9 bodies 1
extrude "Extrude21" cut sketch "Rack Side" against normal up to surface (57 mm away) contours L3 L5 L6 L7 L8 bodies 3
extrude "Extrude22" cut 1 faces at (47, 7.3531, 20) along direction (-1, 0, 0) blind 0.5 on bodies 3 bodies 3
extrude "Extrude23" cut 1 faces at (44.0605, 12.2573, 56.3229) along direction (-0.819152, -0.573576, 0) blind 0.5 on bodies 3 bodies 3
fillet "Fillet1'" radius 0.5 2 edges at (42.14, 15, 54.7594) (42.14, 15, 5.2406) on bodies 3
sketch "Arm Support" plane through (34.2462, 0, 0) normal (-1, 0, 0) x (0, 0, 1)
  line L0 (1.313, 7) -> (1.313, 12)
  line L1 (1.313, 12) -> (3.7092, 12)
  line L2 (3.7092, 12) -> (3.7092, 7)
  line L3 (3.7092, 7) -> (4.7491, 7)
  line L4 (4.7491, 7) -> (4.7491, 12)
  line L5 (4.7491, 12) -> (7.1453, 12)
  line L6 (7.1453, 12) -> (7.1453, 7)
  line L7 (7.1453, 7) -> (8.1852, 7)
  line L8 (8.1852, 7) -> (8.1852, 12)
  line L9 (8.1852, 12) -> (10.5814, 12)
  line L10 (10.5814, 12) -> (10.5814, 7)
  line L11 (10.5814, 7) -> (11.6213, 7)
  line L12 (11.6213, 7) -> (11.6213, 12)
  line L13 (11.6213, 12) -> (14.0175, 12)
  line L14 (14.0175, 12) -> (14.0175, 7)
  line L15 (14.0175, 7) -> (15.0574, 7)
  line L16 (15.0574, 7) -> (15.0574, 12)
  line L17 (15.0574, 12) -> (17.4536, 12)
  line L18 (17.4536, 12) -> (17.4536, 7)
  line L19 (17.4536, 7) -> (18.4935, 7)
  line L20 (18.4935, 7) -> (18.4935, 12)
  line L21 (18.4935, 12) -> (20.8897, 12)
  line L22 (20.8897, 12) -> (20.8897, 7)
  line L23 (20.8897, 7) -> (21.9297, 7)
  line L24 (21.9297, 7) -> (21.9297, 12)
  line L25 (21.9297, 12) -> (24.3259, 12)
  line L26 (24.3259, 12) -> (24.3259, 7)
  line L27 (24.3259, 7) -> (25.3658, 7)
  line L28 (25.3658, 7) -> (25.3658, 12)
  line L29 (25.3658, 12) -> (27.762, 12)
  line L30 (27.762, 12) -> (27.762, 7)
  line L31 (27.762, 7) -> (28.8019, 7)
  line L32 (28.8019, 7) -> (28.8019, 12)
  line L33 (28.8019, 12) -> (31.1981, 12)
  line L34 (31.1981, 12) -> (31.1981, 7)
  line L35 (31.1981, 7) -> (32.238, 7)
  line L36 (32.238, 7) -> (32.238, 12)
  line L37 (32.238, 12) -> (34.6342, 12)
  line L38 (34.6342, 12) -> (34.6342, 7)
  line L39 (34.6342, 7) -> (35.6741, 7)
  line L40 (35.6741, 7) -> (35.6741, 12)
  line L41 (35.6741, 12) -> (38.0703, 12)
  line L42 (38.0703, 12) -> (38.0703, 7)
  line L43 (38.0703, 7) -> (39.1102, 7)
  line L44 (39.1102, 7) -> (39.1102, 12)
  line L45 (39.1102, 12) -> (41.5064, 12)
  line L46 (41.5064, 12) -> (41.5064, 7)
  line L47 (41.5064, 7) -> (42.5464, 7)
  line L48 (42.5464, 7) -> (42.5464, 12)
  line L49 (42.5464, 12) -> (44.9426, 12)
  line L50 (44.9426, 12) -> (44.9426, 7)
  line L51 (44.9426, 7) -> (45.9825, 7)
  line L52 (45.9825, 7) -> (45.9825, 12)
  line L53 (45.9825, 12) -> (48.3787, 12)
  line L54 (48.3787, 12) -> (48.3787, 7)
  line L55 (48.3787, 7) -> (49.4186, 7)
  line L56 (49.4186, 7) -> (49.4186, 12)
  line L57 (49.4186, 12) -> (51.8148, 12)
  line L58 (51.8148, 12) -> (51.8148, 7)
  line L59 (51.8148, 7) -> (52.8547, 7)
  line L60 (52.8547, 7) -> (52.8547, 12)
  line L61 (52.8547, 12) -> (55.2509, 12)
  line L62 (55.2509, 12) -> (55.2509, 7)
  line L63 (55.2509, 7) -> (56.2908, 7)
  line L64 (56.2908, 7) -> (56.2908, 12)
  line L65 (56.2908, 12) -> (58.687, 12)
  line L66 (58.687, 12) -> (58.687, 7)
  line L67 (58.687, 7) -> (60, 7)
  line L68 (60, 7) -> (60, 15)
  line L69 (60, 15) -> (0, 15)
  line L70 (0, 15) -> (0, 7)
  line L71 (0, 7) -> (1.313, 7)
  line L72 (0, 7) -> (0, 17.2)
  line L73 (0, 17.2) -> (0, 67)
  line L74 (0, 26) -> (14.9117, 26) construction
  line L75 (10, 15) -> (0, 25)
  dimension "d197" = 10
  dimension "d198" = 10
  constraint coincident L72 L74.start
  constraint horizontal L74
  constraint coincident L69 L75.start
  constraint coincident L73 L75.end
  measures "d197" distance of L72 L75.start
  measures "d198" distance of L69 L75.end
extrude "Extrude30" add sketch "Arm Support" against normal blind 7 contours L69 L72 L73 L75 bodies 3
copy_body "Body->Comp1" bodies 1 removing the originals makes body 20 in component "Base"
copy_body "Body->Comp2" bodies 3 removing the originals makes body 21 in component "Arm 1"
copy_body "CopyPasteBodies2" bodies 21 makes body 22
move_body "Move2'" bodies 22 to x (-1, 0, 0) y (0, 1, 0) z (0, 0, -1) at (50, 0, 60)
copy_body "Body->Comp4" bodies 22 removing the originals makes body 23 in component "Arm 2"
cylinder "CylinderPrimitive2" cut diameter 9 height -3 placed x (1, 0, 0) y (0, 0, 1) z (0, -1, 0) at (25, 7, 30) bodies 2 in component "Spur Gear (16 teeth)"
ref_plane "WorkPlane2" through (25, -6, 30) normal (0, -1, 0) x (1, 0, 0)
sketch "Handle" plane through (0, -6, 0) normal (0, -1, 0) x (1, 0, 0)
  circle A0 centre (25, 10) radius 2.6
  circle A1 centre (25, 50) radius 2.6
  circle A2 centre (10, 45) radius 2.45
  circle A3 centre (40, 15) radius 2.45
  circle A4 centre (25, 30) radius 2.6
  line L0 (0, 0) -> (50, 0)
  line L1 (50, 0) -> (50, 60)
  line L2 (50, 60) -> (0, 60)
  line L3 (0, 60) -> (0, 0)
  circle A5 centre (25, 30) radius 6
  line L4 (35.3923, 12) -> (45.7846, 30)
  line L5 (45.7846, 30) -> (35.3923, 48)
  line L6 (35.3923, 48) -> (14.6077, 48)
  line L7 (14.6077, 48) -> (4.2154, 30)
  line L8 (4.2154, 30) -> (14.6077, 12)
  line L9 (14.6077, 12) -> (35.3923, 12)
  line L10 (27.3094, 26) -> (29.6188, 30)
  line L11 (29.6188, 30) -> (27.3094, 34)
  line L12 (27.3094, 34) -> (22.6906, 34)
  line L13 (22.6906, 34) -> (20.3812, 30)
  line L14 (20.3812, 30) -> (22.6906, 26)
  line L15 (22.6906, 26) -> (27.3094, 26)
  line L16 (25, 30) -> (40.5885, 21) construction
  spline S0 degree 2 poles (35.3923, 12) (34.2376, 24.6667) (45.7846, 30) knots 0 0 0 2.204037 2.204037 2.204037
  spline S1 degree 2 poles (45.7846, 30) (34.2376, 35.3333) (35.3923, 48) knots 0 0 0 2.204037 2.204037 2.204037
  spline S2 degree 2 poles (35.3923, 48) (25, 40.6667) (14.6077, 48) knots 0 0 0 2.204037 2.204037 2.204037
  spline S3 degree 2 poles (14.6077, 48) (15.7624, 35.3333) (4.2154, 30) knots 0 0 0 2.204037 2.204037 2.204037
  spline S4 degree 2 poles (4.2154, 30) (15.7624, 24.6667) (14.6077, 12) knots 0 0 0 2.204037 2.204037 2.204037
  spline S5 degree 2 poles (14.6077, 12) (25, 19.3333) (35.3923, 12) knots 0 0 0 2.204037 2.204037 2.204037
  point P0 (25, 30)
  point P1 (25, 30)
  dimension "d153" = 12
  dimension "d154" = 18
  dimension "d155" = 4
  dimension "d194" = 360
  constraint coincident P1 P0
  constraint midpoint L4 L16.end
  measures "d153" diameter of A5
  measures "d154" distance of P1 L9
  measures "d155" distance of P1 L15
extrude "Extrude27" add sketch "Handle" against normal blind 5 separate body contours S0 S1 S2 S3 S4 S5 | A5 | L10 L11 L12 L13 L14 L15 makes body 24
extrude "Extrude28" add sketch "Handle" against normal blind 6 contours A5 | L10 L11 L12 L13 L14 L15 bodies 24
extrude "Extrude29" add sketch "Handle" along normal blind 3 contours S0 S1 S2 S3 S4 S5 | A5 bodies 24
copy_body "Body->Comp5" bodies 24 removing the originals makes body 25 in component "Handle"
fillet "Fillet1''" radius 3 6 edges at (35.3923, -5, 48) (45.7846, -5, 30) (14.6077, -5, 48) (4.2154, -5, 30) (35.3923, -5, 12) (14.6077, -5, 12) on bodies 25 in component "Handle"
component "Spur Gear (16 teeth)" placed x (1, 0, 0) y (0, 1, 0) z (0, 0, 1) at (0, 0, 0)
component "Base" placed x (1, 0, 0) y (0, 1, 0) z (0, 0, 1) at (0, 0, 0)
component "Arm 1" placed x (1, 0, 0) y (0, 1, 0) z (0, 0, 1) at (0, 0, 0)
component "Arm 2" placed x (1, 0, 0) y (0, 1, 0) z (0, 0, 1) at (0, 0, 0)
component "Handle" placed x (1, 0, 0) y (0, 1, 0) z (0, 0, 1) at (0, 0, 0)
equation "diametricalpitch = 16 mm"
equation "spurteeth = 16"
equation "pressureangle = 20 deg"
equation "thickness = 5 mm"
equation "pitchcirclediam = ( spurteeth / diametricalpitch * 1 mm ) * 10 mm"
equation "backlash = 0.05 mm"